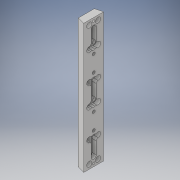
# Autodesk Inventor part: dovetail2
Saved by Autodesk Inventor 2019.4 (Build 234330000, 330)
## iProperties
Created: 2020-08-31
Part Number: dovetail2
Material: Ogólny
Document SubType Name: Modeling
Designer: barto
Density: 1 g/cm^3
Appearance: Domyślna
Author: barto
Autodesk Inventor part; units mm, degrees
ref_plane "YZ Plane" through (0, 0, 0) normal (1, 0, 0) x (0, 1, 0)
ref_plane "XZ Plane" through (0, 0, 0) normal (0, 1, 0) x (-1, 0, 0)
sketch "Szkic1" plane through (0, 0, 0) normal (0, 1, 0) x (-1, 0, 0)
  line L0 (0, 0) -> (0, -43.18)
  line L1 (0, -43.18) -> (15.875, -38.9263)
  line L2 (0, -43.18) -> (16.435, -43.18) construction
  line L3 (0, 0) -> (15.875, -4.2537)
  line L4 (0, 0) -> (18.9194, 0) construction
  line L5 (15.875, -21.59) -> (15.875, -4.2537)
  line L6 (15.875, -21.59) -> (15.875, -38.9263)
  dimension "d0" = 43.18
  dimension "d2" = 15
  dimension "d3" = 15
  dimension "d4" = 15.875
  constraints: 14 end point, 3 vertical, 2 horizontal, 1 equal length
  measures "d0" distance of L0.start L0.end
  measures "d2" angle of L2 L1
  measures "d3" angle of L3 L4
  measures "d4" distance between parallel lines of L0 L6
extrude "Wyciągnięcie proste1" add sketch "Szkic1" along normal blind 279.4
sketch "Szkic2" plane through (0, 0, 0) normal (1, 0, 0) x (0, 0, -1)
  line L0 (0, 0) -> (43.18, 0) projected
  line L1 (0, 279.4) -> (43.18, 279.4) projected
  line L2 (43.18, 0) -> (43.18, 279.4) projected
  line L3 (0, 0) -> (0, 279.4) projected
  point P0 (12.065, 9.525)
  point P1 (12.065, 55.245)
  point P2 (12.065, 224.155)
  point P3 (12.065, 269.875)
  point P4 (31.115, 269.875)
  point P5 (31.115, 224.155)
  point P6 (31.115, 55.245)
  point P7 (31.115, 9.525)
  point P8 (31.115, 162.56)
  point P9 (31.115, 116.84)
  point P10 (12.065, 162.56)
  point P11 (12.065, 116.84)
  dimension "d7" = 45.72
  dimension "d9" = 45.72
  dimension "d10" = 9.525
  dimension "d12" = 19.05
  dimension "d13" = 19.05
  dimension "d14" = 19.05
  dimension "d15" = 19.05
  dimension "d18" = 12.065
  dimension "d19" = 12.065
  dimension "d20" = 12.065
  dimension "d21" = 12.065
  dimension "d48" = 9.525
  dimension "d49" = 45.72
  dimension "d51" = 45.72
  dimension "d103" = 9.525
  dimension "d104" = 9.525
  dimension "d107" = 61.595
  dimension "d108" = 61.595
  dimension "d109" = 61.595
  dimension "d110" = 61.595
  measures "d7" distance of point (12.065, 55.245) point (12.065, 9.525)
  measures "d9" distance of point (12.065, 269.875) point (12.065, 224.155)
  measures "d10" distance from line of L0 point (12.065, 9.525)
  measures "d12" distance of point (12.065, 9.525) point (31.115, 9.525)
  measures "d13" distance of point (12.065, 55.245) point (31.115, 55.245)
  measures "d14" distance of point (12.065, 224.155) point (31.115, 224.155)
  measures "d15" distance of point (12.065, 269.875) point (31.115, 269.875)
  measures "d18" distance from line of L3 point (12.065, 269.875)
  measures "d19" distance from line of L3 point (12.065, 224.155)
  measures "d20" distance from line of L3 point (12.065, 55.245)
  measures "d21" distance from line of L3 point (12.065, 9.525)
  measures "d48" distance from line of L0 point (31.115, 9.525)
  measures "d49" distance of point (31.115, 224.155) point (31.115, 269.875)
  measures "d51" distance of point (31.115, 9.525) point (31.115, 55.245)
  measures "d103" distance from line of L1 point (31.115, 269.875)
  measures "d104" distance from line of L1 point (12.065, 269.875)
  measures "d107" distance of point (31.115, 162.56) point (31.115, 224.155)
  measures "d108" distance of point (31.115, 55.245) point (31.115, 116.84)
  measures "d109" distance of point (12.065, 224.155) point (12.065, 162.56)
  measures "d110" distance of point (12.065, 55.245) point (12.065, 116.84)
hole "Otwór1" at (0, 9.525, -12.065) at (0, 55.245, -12.065) at (0, 224.155, -12.065) at (0, 269.875, -12.065) at (0, 269.875, -31.115) at (0, 224.155, -31.115) at (0, 55.245, -31.115) at (0, 9.525, -31.115) at (0, 162.56, -31.115) at (0, 116.84, -31.115) at (0, 116.84, -12.065) at (0, 162.56, -12.065) direction (-1, 0, 0) diameter 6.756 depth 30 tip angle 118 counterbore diameter 11.113 counterbore depth 8.89 clearance for "Wkręt z łbem walcowym gniazdowym" size "1/4" standard "ANSI Gwinty cal zunifikowane"
sketch "Szkic3" plane through (-15.875, 0, -38.9263) normal (-1, 0, 0) x (0, 0, 1)
  line L0 (34.6726, 0) -> (34.6726, 279.4) projected
  line L1 (0, 0) -> (0, 279.4) projected
  line L2 (0, 279.4) -> (34.6726, 279.4) projected
  point P0 (38.9263, 0)
  point P1 (17.3366, 211.4)
  point P2 (17.3366, 176.4)
  dimension "d29" = 17.336
  dimension "d31" = 17.336
  dimension "d34" = 35
  dimension "d35" = 68
  measures "d29" distance from line of L0 point (17.337, 211.4)
  measures "d31" distance from line of L0 point (17.337, 176.4)
  measures "d34" distance of point (17.337, 211.4) point (17.337, 176.4)
  measures "d35" distance from line of L2 point (17.337, 211.4)
hole "Otwór2" at (-15.875, 211.4, -21.5897) at (-15.875, 176.4, -21.5897) direction (1, 0, 0) diameter 6.401 depth 22.931 tip angle 118 thread size "5/16-18 UNC" class "2B" standard "ANSI Unified Screw Threads"
sketch "Szkic4" plane through (-15.875, 0, -38.9263) normal (-1, 0, 0) x (0, 0, 1)
  line L0 (0, 0) -> (0, 279.4) projected
  line L1 (34.6726, 0) -> (34.6726, 279.4) projected
  circle A0 centre (26.8613, 224.155) radius 5.5565 projected
  circle A1 centre (26.8613, 55.245) radius 3.378 projected
  circle A2 centre (7.8113, 55.245) radius 3.378 projected
  arc A3 (20.7143, 55.245) -> (13.9583, 55.245) centre (17.3363, 55.245) ccw
  arc A4 (13.9583, 19.456) -> (20.7143, 19.456) centre (17.3363, 19.456) ccw
  line L2 (20.7143, 55.245) -> (20.7143, 19.456)
  line L3 (13.9583, 19.456) -> (13.9583, 55.245)
  line L4 (0, 0) -> (34.6726, 0) projected
  line L5 (0, 279.4) -> (34.6726, 279.4) projected
  arc A5 (20.7143, 259.944) -> (13.9583, 259.944) centre (17.3363, 259.944) ccw
  arc A6 (13.9583, 224.155) -> (20.7143, 224.155) centre (17.3363, 224.155) ccw
  line L6 (20.7143, 259.944) -> (20.7143, 224.155)
  line L7 (13.9583, 224.155) -> (13.9583, 259.944)
  circle A7 centre (7.8113, 116.84) radius 5.5565 projected
  circle A8 centre (26.8613, 116.84) radius 3.378 projected
  circle A9 centre (26.8613, 162.56) radius 3.378 projected
  circle A10 centre (7.8113, 162.56) radius 3.378 projected
  arc A11 (13.9583, 116.84) -> (20.7143, 116.84) centre (17.3363, 116.84) ccw
  arc A12 (20.7143, 162.56) -> (13.9583, 162.56) centre (17.3363, 162.56) ccw
  line L8 (13.9583, 116.84) -> (13.9583, 162.56)
  line L9 (20.7143, 162.56) -> (20.7143, 116.84)
  line L10 (13.3678, 116.84) -> (13.9583, 116.84)
  point P0 (38.9263, 0)
  point P1 (17.3363, 259.944)
  dimension "d56" = 6.756
  dimension "d57" = 6.756
  dimension "d66" = 35.789
  dimension "d67" = 35.789
  dimension "d68" = 0
  dimension "d87" = 19.456
  dimension "d90" = 19.456
  dimension "d91" = 6.756
  dimension "d92" = 6.756
  dimension "d93" = 35.789
  dimension "d94" = 35.789
  constraints: 14 end point, 12 point on circle, 6 centre point, 2 tangent, 1 horizontal, 1 horizontal alignment, 1 other
  measures "d56" diameter of A3
  measures "d57" diameter of A4
  measures "d66" distance of L2.start L2.end
  measures "d67" distance of L3.start L3.end
  measures "d68" vertical distance of A1.centre A3.centre
  measures "d87" distance from line of L4 A4.centre
  measures "d90" distance from line of L5 point (17.336, 259.944)
  measures "d91" diameter of A5
  measures "d92" diameter of A6
  measures "d93" distance of L6.start L6.end
  measures "d94" distance of L7.start L7.end
sketch "Szkic8" plane through (-15.875, 0, -38.9263) normal (-1, 0, 0) x (0, 0, 1)
  arc A0 (13.9583, 19.456) -> (20.7143, 19.456) centre (17.3363, 19.456) ccw projected
  line L0 (17.3363, 19.456) -> (17.3363, 202.652)
  line L1 (17.3363, 19.456) -> (17.3363, -13.8574)
  line L2 (0, 279.4) -> (34.6726, 279.4) projected
  line L3 (0, 0) -> (34.6726, 0) projected
  point P0 (38.9263, 0)
  point P1 (17.3363, 6.5)
  point P2 (17.3363, 272.9)
  dimension "d78" = 6.5
  dimension "d79" = 6.5
  constraints: 4 end point, 2 point on line, 2 vertical
  measures "d78" distance from line of L2 point (17.336, 272.9)
  measures "d79" distance from line of L3 point (17.336, 6.5)
hole "Otwór3" at (-15.875, 6.5, -21.59) at (-15.875, 272.9, -21.59) direction (1, 0, 0) diameter 4.978 depth 19.05 tip angle 118 thread size "1/4-20 UNC" class "2B" standard "ANSI Unified Screw Threads"
extrude "Wyciągnięcie proste5" cut sketch "Szkic4" against normal blind 25 contours L2 A4 L3 A3 | L6 A6 L7 A5 | L8 A12 L9 A11
sketch "Szkic7" plane through (0, 0, 0) normal (1, 0, 0) x (0, 0, -1)
  arc A0 (16.0335, 19.456) -> (27.1465, 19.456) centre (21.59, 19.456) ccw
  arc A1 (27.1465, 55.245) -> (16.0335, 55.245) centre (21.59, 55.245) ccw
  line L0 (16.0335, 19.456) -> (16.0335, 55.245)
  line L1 (27.1465, 19.456) -> (27.1465, 55.245)
  arc A2 (16.0335, 224.155) -> (27.1465, 224.155) centre (21.59, 224.155) ccw
  arc A3 (27.1465, 259.944) -> (16.0335, 259.944) centre (21.59, 259.944) ccw
  line L2 (27.1465, 259.944) -> (27.1465, 224.155)
  line L3 (16.0335, 224.155) -> (16.0335, 259.944)
  arc A4 (24.968, 162.56) -> (18.212, 162.56) centre (21.59, 162.56) ccw projected
  arc A5 (27.1465, 162.56) -> (16.0335, 162.56) centre (21.59, 162.56) ccw
  arc A6 (18.212, 116.84) -> (24.968, 116.84) centre (21.59, 116.84) ccw projected
  arc A7 (16.0335, 116.84) -> (27.1465, 116.84) centre (21.59, 116.84) ccw
  line L4 (16.0335, 116.84) -> (16.0335, 162.56)
  line L5 (27.1465, 162.56) -> (27.1465, 116.84)
  point P0 (0, 0)
  dimension "d71" = 11.113
  dimension "d72" = 11.113
  dimension "d111" = 11.113
  dimension "d112" = 11.113
  constraints: 12 end point, 12 point on circle, 6 centre point, 4 tangent, 2 coincident, 2 parallel, 1 vertical
  measures "d71" diameter of A0
  measures "d72" diameter of A1
  measures "d111" diameter of A5
  measures "d112" diameter of A7
extrude "Wyciągnięcie proste6" cut sketch "Szkic7" against normal blind 8.89
ref_plane "Płaszczyzna konstrukcyjna2" through (0, 139.7, 0) normal (0, -1, 0) x (1, 0, 0)
mirror "Odbij1" about plane through (0, 139.7, 0) normal (0, -1, 0) of "Otwór2"
fillet "Zaokrąglenie2" radius 4 16 edges at (-4.445, 58.1074, -16.8275) (-4.445, 58.1074, -26.3525) (-4.445, 51.3558, -16.0335) (-4.445, 51.3558, -27.1465) (-4.445, 228.0442, -16.0335) (-4.445, 228.0442, -27.1465) (-4.445, 221.2926, -16.8275) (-4.445, 221.2926, -26.3525) (-4.445, 158.6708, -16.0335) (-4.445, 120.7292, -16.0335) (-4.445, 158.6708, -27.1465) (-4.445, 120.7292, -27.1465) (-4.445, 165.4224, -16.8275) (-4.445, 165.4224, -26.3525) (-4.445, 113.9776, -16.8275) (-4.445, 113.9776, -26.3525)
equation "\"d9\" = d7"
equation "\"d13\" = d12"
equation "\"d14\" = d13"
equation "\"d15\" = d14"
equation "\"d48\" = d10"
equation "\"d49\" = d9"
equation "\"d51\" = d7"
equation "\"d103\" = d10"
equation "\"d104\" = d103"
equation "\"d108\" = d107"
equation "\"d109\" = d107"
equation "\"d110\" = d108"
equation "\"d31\" = d29"
equation "\"d67\" = d66"
equation "\"d90\" = d87"
equation "\"d94\" = d93"
